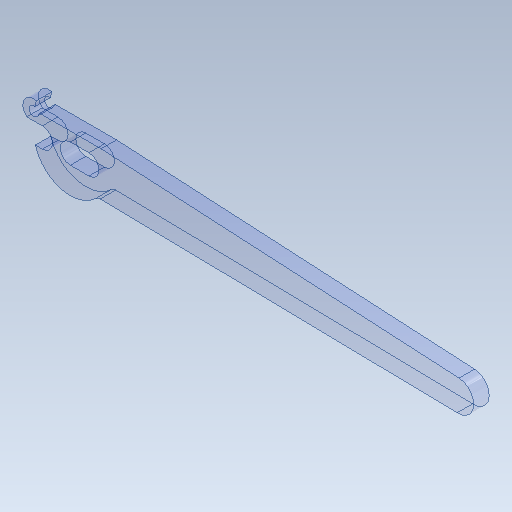
# Autodesk Inventor part: Wing2
Saved by Autodesk Inventor 2020.2 (Build 242310000, 310)
## iProperties
Created: 2020-04-12
Part Number: Wing2
Material: ポリカーボネート、クリア
Document SubType Name: Modeling
Designer: aoyama
Density: 1.2 g/cm^3
Appearance: トロピカル 青
Mass: 10.1133 g
Surface Area: 51.7953 cm^2
Volume: 8.42772 cm^3
Author: aoyama
Autodesk Inventor part; units mm, degrees
ref_plane "YZ Plane" through (0, 0, 0) normal (1, 0, 0) x (0, 1, 0)
ref_plane "XZ Plane" through (0, 0, 0) normal (0, 1, 0) x (-1, 0, 0)
ref_plane "XY Plane" through (0, 0, 0) normal (0, 0, 1) x (1, 0, 0)
sketch "スケッチ1" plane through (0, 0, 0) normal (0, 0, 1) x (1, 0, 0)
  line L0 (0, 0) -> (6, 0) construction
  line L1 (0, -3.25) -> (6, -3.25)
  line L2 (6, 3.25) -> (0, 3.25)
  arc A0 (0, 3.25) -> (0, -3.25) centre (0, 0) ccw
  arc A1 (6, -3.25) -> (6, 3.25) centre (6, 0) ccw
  line L3 (-15, 0) -> (-9, 0) construction
  line L4 (-9, 3.25) -> (-15, 3.25)
  arc A2 (-15, 3.25) -> (-18.25, 0) centre (-15, 0) ccw
  arc A3 (-9, -3.25) -> (-9, 3.25) centre (-9, 0) ccw
  line L5 (-9, 0) -> (0, 0)
  circle A4 centre (-15, 0) radius 3.25 construction
  circle A5 centre (2.6047, -14.7721) radius 3.25
  line L6 (0, 0) -> (2.6047, -14.7721) construction
  arc A6 (-11.2916, -3.25) -> (2.0404, -11.5715) centre (0, 0) ccw
  line L7 (0, 0) -> (125.4, 0)
  line L8 (125.262, -9.9907) -> (5.461, -13.2216)
  line L9 (-11.2916, -3.25) -> (-9, -3.25)
  arc A7 (-11.75, 0) -> (-11.2916, -3.25) centre (0, 0) ccw
  arc A8 (2.0404, -11.5715) -> (-11.75, 0) centre (0, 0) ccw
  line L10 (9.9117, 6.3104) -> (125.4, 0)
  line L11 (-9.9117, 6.3104) -> (9.9117, 6.3104)
  line L12 (-15, 6.3104) -> (-15, 0) construction
  circle A9 centre (125.1272, -4.9926) radius 5
  line L13 (8.7592, -7.832) -> (125.262, -9.9907)
  circle A10 centre (-11.8389, 5.95) radius 1.5
  arc A11 (-13.6588, 2.9604) -> (-8.835, 7.7463) centre (-11.8389, 5.95) ccw
  arc A12 (-8.835, 7.7463) -> (-10.9368, 9.3317) centre (-11.8389, 5.95) ccw construction
  arc A13 (-14.066, 3.25) -> (-13.6588, 2.9604) centre (-11.8389, 5.95) ccw
  line L14 (-11.8389, 5.95) -> (-10.9368, 9.3317)
  arc A14 (-10.9368, 9.3317) -> (-14.066, 3.25) centre (-11.8389, 5.95) ccw
  point P0 (3, 0)
  point P1 (-12, 0)
  point P2 (2.0404, -11.5715)
  point P3 (124.8544, 0)
  point P4 (11.75, 0)
  point P5 (124.8073, -9.9823)
  point P6 (-11.2916, 3.25)
  point P7 (-10.4987, 5.2764)
  point P8 (-11.4523, 7.3993)
  point P9 (-11.488, 2.4676)
  dimension "d7" = 6.5
  dimension "d0" = 6.5
  dimension "d1" = 6
  dimension "d3" = 6.5
  dimension "d4" = 6
  dimension "d5" = 15
  dimension "d6" = 6.5
  dimension "d8" = 15
  dimension "d9" = 100
  dimension "d11" = 125.4
  dimension "d18" = 10
  dimension "d26" = 3
  dimension "d27" = 2
  dimension "d28" = 1.2
  constraints: 34 end point, 31 point on circle, 14 centre point, 12 tangent, 5 horizontal, 3 coincident, 3 point on line, 2 midpoint, 2 parallel, 1 vertical, 3 other
  measures "d0" diameter of A1
  measures "d1" distance of L0.start L0.end
  measures "d3" diameter of A3
  measures "d4" distance of L3.start L3.end
  measures "d5" distance of L3.start point (0, 0)
  measures "d6" diameter of A4
  measures "d8" distance of L6.end point (0, 0)
  measures "d9" angle of L6 L5
  measures "d11" distance of L0.start L7.end
  measures "d18" diameter of A9
  measures "d26" diameter of A10
  measures "d27" radial gap between concentric circles of A10 A11
  measures "d28" distance edge to line of A10 L4
extrude "押し出し1" add sketch "スケッチ1" along normal blind 5 contours L1 A1 L7 A8 A6 L9 A3 L5 A0 | L5 A3 L4 A11 L11 A8 L7 A1 L2 A0 | A8 L10 A9 L7 | A9 L7 | L7 A9 L13 A8 | A9 L7 | L4 A8 L11 A11 | L4 A14 L14 A10 A8
fillet "フィレット2" radius 2 1 edges at (8.7592, -7.832, 2.5)
